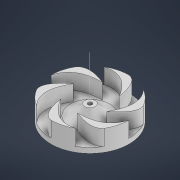
# Autodesk Inventor part: Fan2
Saved by Autodesk Inventor 2022 (Build 260153000, 153)
## iProperties
Created: 2022-06-25
Part Number: Fan2
Material: 一般
Document SubType Name: Modeling
Designer: neko2
Density: 1 g/cm^3
Appearance: 既定
Author: neko2
Autodesk Inventor part; units mm, degrees
ref_plane "YZ Plane" through (0, 0, 0) normal (1, 0, 0) x (0, 1, 0)
ref_plane "XZ Plane" through (0, 0, 0) normal (0, 1, 0) x (-1, 0, 0)
ref_plane "XY Plane" through (0, 0, 0) normal (0, 0, 1) x (1, 0, 0)
sketch "スケッチ1" plane through (0, 0, 0) normal (0, 1, 0) x (-1, 0, 0)
  circle A0 centre (0, 0) radius 7.5
  dimension "d0" = 15
  constraints: 1 centre point, 1 coincident
  measures "d0" diameter of A0
extrude "押し出し1" add sketch "スケッチ1" along normal blind 1
sketch "スケッチ2" plane through (0, 1, 0) normal (0, 1, 0) x (1, 0, 0)
  circle A0 centre (0, 0) radius 7.5 projected
  line L0 (0, 0) -> (-7.5, 0)
  line L1 (0, 0) -> (-1.3681, 3.7588)
  line L2 (-7.5, 0) -> (-6.4952, 3.75) construction
  line L3 (-6.4952, 3.75) -> (-1.3681, 3.7588) construction
  spline S0 degree 2 poles (-7.5, 0) (-6.4952, 3.75) (-1.3681, 3.7588) knots 1 1 1 2 2 2
  line L4 (-6.4952, 3.75) -> (-5.3033, 5.3033) construction
  line L5 (-5.3033, 5.3033) -> (-1.3681, 3.7588) construction
  spline S1 degree 2 poles (-6.4952, 3.75) (-5.3033, 5.3033) (-1.3681, 3.7588) knots 1 1 1 2 2 2
  line L6 (0, 0) -> (-5.3033, 5.3033)
  line L7 (-6.4952, 3.75) -> (0, 0)
  point P0 (-6.4952, 3.75)
  dimension "d5" = 70
  dimension "d14" = 4
  dimension "d18" = 25
  dimension "d19" = 15
  constraints: 8 end point, 3 coincident, 3 point on circle, 1 horizontal, 6 other
  measures "d5" angle of L0 L1
  measures "d14" distance of L0.start L1.end
  measures "d18" angle of L1 L6
  measures "d19" angle of L7 L6
extrude "押し出し2" add sketch "スケッチ2" along normal blind 3 contours A0 L7 S0 | S1 L6 S0 L7 | S1 S0 L6
pattern_circular "円形状パターン1" count 6 over 360 about axis through (0, 1, 0) along (0, 1, 0) of "押し出し2"
sketch "スケッチ4" plane through (0, 1, 0) normal (0, 1, 0) x (1, 0, 0)
  circle A0 centre (0, 0) radius 1
  dimension "d20" = 2
  constraints: 1 centre point, 1 coincident
  measures "d20" diameter of A0
extrude "押し出し4" add sketch "スケッチ4" along normal blind 2 and the other way blind 2
fillet "フィレット1" radius 3 1 edges at (-1, 1, 0)
sketch "スケッチ5" plane through (0, 3, 0) normal (0, 1, 0) x (1, 0, 0)
  circle A0 centre (0, 0) radius 0.4
  dimension "d24" = 0.8
  constraints: 1 centre point, 1 coincident
  measures "d24" diameter of A0
extrude "押し出し5" cut sketch "スケッチ5" against normal through all
fillet "フィレット2" radius 2 1 edges at (-1, 0, 0)
